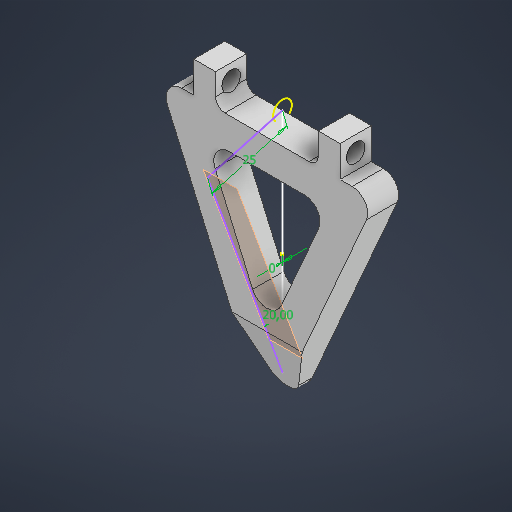
# Autodesk Inventor part: trojúhleník_closer
Saved by Autodesk Inventor 2026 (Build 300175050, 175E)
## iProperties
Created: 2026-02-24
Part Number: trojúhleník_closer
Material: Všeobecné
Document SubType Name: Modeling
Designer: marti
Density: 1 g/cm^3
Appearance: Výchozí
Author: marti
Autodesk Inventor part; units mm, degrees
ref_plane "XZ Plane" through (0, 0, 0) normal (0, 1, 0) x (-1, 0, 0)
ref_plane "XY Plane" through (0, 0, 0) normal (0, 0, 1) x (1, 0, 0)
sketch "Náčrt1" plane through (0, 0, 0) normal (0, 0, 1) x (1, 0, 0)
  line L0 (-35, 35) -> (35, 35)
  line L1 (-35, 35) -> (0, -45)
  line L2 (0, -45) -> (35, 35)
  line L3 (0, 51) -> (0, -61) projected
  line L4 (-49, 0) -> (49, 0) projected
  line L5 (19.7098, 25) -> (-19.7098, 25)
  line L6 (-19.7098, 25) -> (0, -20.0511)
  line L7 (0, -20.0511) -> (19.7098, 25)
  point P0 (0, 0)
  dimension "d3" = 70
  dimension "d36" = 80
  dimension "d37" = 35
  dimension "d38" = 10
  constraints: 12 end point, 1 parallel, 1 point on line, 1 symmetric about line, 2 other
  measures "d3" distance of L0.start L0.end
  measures "d36" distance from line of L0 L1.end
  measures "d37" distance between parallel lines of L0 L4
  measures "d38" distance between parallel lines of L2 L7
extrude "Vysunutí1" add sketch "Náčrt1" along normal mid plane 10 contours L0 L3 L5 L6 L4 L1 | L0 L2 L4 L7 L5 L3 | L4 L6 L3 L1 | L3 L7 L4 L2
fillet "Zaoblení1" radius 5 6 edges at (-35, 35, 0) (35, 35, 0) (0, -45, 0) (0, -20.0511, 0) (-19.7098, 25, 0) (19.7098, 25, 0)
ref_plane "Pracovní rovina1" through (20, 0, 0) normal (1, 0, 0) x (0, 1, 0)
ref_plane "Pracovní rovina2" through (-20, 0, 0) normal (1, 0, 0) x (0, 1, 0)
sketch "Náčrt3" plane through (20, 0, 0) normal (1, 0, 0) x (0, 1, 0)
  line L0 (45, -5) -> (30, -5)
  line L1 (30, -5) -> (30, 5)
  line L2 (30, 5) -> (45, 5)
  line L3 (45, 5) -> (45, -5)
  line L4 (35, 5) -> (35, -5) projected
  point P0 (0, 0)
  dimension "d18" = 15
  dimension "d19" = 10
  dimension "d20" = 10
  constraints: 8 end point, 2 parallel, 1 horizontal, 1 perpendicular
  measures "d18" distance of L1.end L2.end
  measures "d19" distance of L0.end L1.end
  measures "d20" distance between parallel lines of L4 L3
sketch "Náčrt4" plane through (-20, 0, 0) normal (1, 0, 0) x (0, 1, 0)
  line L0 (45, -5) -> (45, 5) projected
  line L1 (35, -5) -> (45, -5) projected
  line L2 (45, 5) -> (35, 5) projected
  line L3 (35, -5) -> (27.9959, -5) projected
  line L4 (27.9959, -5) -> (27.9959, 5) projected
  line L5 (27.9959, 5) -> (35, 5) projected
  line L6 (35, 5) -> (35, -5) projected
  line L7 (45, -5) -> (35, -5)
  line L8 (35, -5) -> (35, 5)
  line L9 (35, 5) -> (45, 5)
  line L10 (45, 5) -> (45, -5)
  point P0 (0, 0)
  constraints: 8 end point, 2 parallel, 1 horizontal, 1 perpendicular
extrude "Vysunutí2" add sketch "Náčrt4" along normal mid plane 7
extrude "Vysunutí3" add sketch "Náčrt3" along normal mid plane 7
fillet "Zaoblení2" radius 3 2 edges at (16.5, 35, 0) (-16.5, 35, 0)
sketch "Náčrt5" plane through (23.5, 0, 0) normal (1, 0, 0) x (0, 0, -1)
  line L0 (5, 35) -> (5, 45) projected
  line L1 (5, 45) -> (-5, 45) projected
  line L2 (-5, 45) -> (-5, 35) projected
  line L3 (5, 35) -> (-5, 35) projected
  point P0 (0, 0)
  point P1 (0, 40)
hole "Díra1" at (23.5, 40, 0) direction (-1, 0, 0) diameter 6 end through all
sketch "Náčrt8" plane through (0, 0, 0) normal (1, 0, 0) x (0, 1, 0)
  arc A0 (38, -2.2361) -> (38, 2.2361) centre (40, 0) ccw projected
  line L0 (-32.8803, 0) -> (40, 0)
  line L1 (40, 0) -> (33.2745, 24.0784)
  line L2 (-32.8803, 0) -> (33.2745, 24.0784)
  point P0 (0, 0)
  dimension "d44" = 25
  dimension "d45" = 20
  dimension "d46" = 0
  constraints: 6 end point
  measures "d44" distance of L0.end L1.end
  measures "d45" angle of L2 L0
  measures "d46" distance from line of point (0, 0) L0
ref_plane "Pracovní rovina5" through (0, -19.1429, 5) normal (0, -0.3420201, 0.9396926) x (1, 0, 0)
sketch "Náčrt9" plane through (0, -19.1429, 5) normal (0, -0.3420201, 0.9396926) x (1, 0, 0)
  line L0 (-53.9277, 46.4461) -> (54.4181, 46.4461)
  line L1 (54.4181, 46.4461) -> (54.4181, -37.1249)
  line L2 (54.4181, -37.1249) -> (-53.9277, -37.1249)
  line L3 (-53.9277, -37.1249) -> (-53.9277, 46.4461)
  point P0 (0, 16.2783)
  constraints: 8 end point, 2 parallel, 1 horizontal, 1 perpendicular
extrude "Vysunutí6" cut sketch "Náčrt9" along normal blind 10
